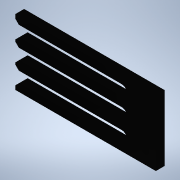
# Autodesk Inventor part: SampleMountFingers
Saved by Autodesk Inventor 2022.2 (Build 262287000, 287)
## iProperties
Created: 2021-09-07
Part Number: SampleMountFingers
Material: Aluminum 6061
Document SubType Name: Modeling
Designer: Timo
Density: 2.7 g/cm^3
Appearance: Anodized - Black
Author: Timo
Autodesk Inventor part; units mm, degrees
ref_plane "YZ Plane" through (0, 0, 0) normal (1, 0, 0) x (0, 1, 0)
ref_plane "XZ Plane" through (0, 0, 0) normal (0, 1, 0) x (-1, 0, 0)
ref_plane "XY Plane" through (0, 0, 0) normal (0, 0, 1) x (1, 0, 0)
sketch "Sketch1" plane through (0, 0, 0) normal (0, 0, 1) x (1, 0, 0)
  line L0 (0, 0) -> (-60, 0) construction
  line L1 (0, 3.1) -> (-60, 3.1)
  line L2 (-60, -3.1) -> (0, -3.1)
  arc A0 (0, -3.1) -> (0, 3.1) centre (0, 0) ccw
  arc A1 (-60, 3.1) -> (-60, -3.1) centre (-60, 0) ccw
  line L3 (0, 11.2) -> (-60, 11.2) construction
  line L4 (0, 14.3) -> (-60, 14.3)
  line L5 (-60, 8.1) -> (0, 8.1)
  arc A2 (0, 8.1) -> (0, 14.3) centre (0, 11.2) ccw
  arc A3 (-60, 14.3) -> (-60, 8.1) centre (-60, 11.2) ccw
  line L6 (0, -11.2) -> (-60, -11.2) construction
  line L7 (0, -8.1) -> (-60, -8.1)
  line L8 (-60, -14.3) -> (0, -14.3)
  arc A4 (0, -14.3) -> (0, -8.1) centre (0, -11.2) ccw
  arc A5 (-60, -8.1) -> (-60, -14.3) centre (-60, -11.2) ccw
  line L9 (7.3, -3.9) -> (-7.3, -3.9) construction
  line L10 (-7.3, -3.9) -> (-7.3, -18.5) construction
  line L11 (-7.3, -18.5) -> (7.3, -18.5) construction
  line L12 (7.3, -18.5) -> (7.3, -3.9) construction
  line L13 (7.3, 3.9) -> (-7.3, 3.9) construction
  line L14 (-7.3, 3.9) -> (-7.3, 18.5) construction
  line L15 (-7.3, 18.5) -> (7.3, 18.5) construction
  line L16 (7.3, 18.5) -> (7.3, 3.9) construction
  line L17 (-7.3, -3.9) -> (7.3, -18.5) construction
  line L18 (7.3, -3.9) -> (-7.3, -18.5) construction
  line L19 (-7.3, 18.5) -> (7.3, 3.9) construction
  line L20 (7.3, 18.5) -> (-7.3, 3.9) construction
  line L21 (0, -25.9) -> (0, 25.9) construction
  line L22 (-60, 18.5) -> (7.3, 18.5)
  line L23 (7.3, 18.5) -> (7.3, -18.5)
  line L24 (7.3, -18.5) -> (-60, -18.5)
  line L25 (-60, -18.5) -> (-60, 18.5)
  line L26 (7.3, 18.5) -> (19.3, 18.5)
  line L27 (19.3, 18.5) -> (19.3, -18.5)
  line L28 (19.3, -18.5) -> (7.3, -18.5)
  line L29 (7.3, -18.5) -> (7.3, 18.5)
  point P0 (-30, 0)
  point P1 (-30, 11.2)
  point P2 (-30, -11.2)
  point P3 (0, -11.2)
  dimension "d0" = 6.2
  dimension "d1" = 14.6
  dimension "d2" = 14.6
  dimension "d5" = 60
  dimension "d11" = 11.2
  dimension "d12" = 5
  dimension "d13" = 5
  dimension "d17" = 37
  dimension "d18" = 12
  constraints: 64 end point, 13 parallel, 12 point on circle, 12 tangent, 6 centre point, 6 midpoint, 5 horizontal, 5 perpendicular, 4 equal length, 3 point on line, 2 equal radius
  measures "d0" diameter of A1
  measures "d1" distance of L11.end L10.end
  measures "d2" distance of L10.end L9.end
  measures "d5" distance of L6.start L6.end
  measures "d11" distance between parallel lines of L0 L3
  measures "d12" distance between parallel lines of L7 L2
  measures "d13" distance between parallel lines of L1 L5
  measures "d17" distance of L15.end L11.end
  measures "d18" distance of L15.end L26.end
extrude "Extrusion1" add sketch "Sketch1" along normal blind 5 contours L1 L25 L5 A2 L4 L22 L23 L24 L8 A4 L7 L2 A0 | L26 L27 L28 L23
chamfer "Chamfer1" distance 2 angle 45 6 edges at (-60, 14.3, 2.5) (-60, 8.1, 2.5) (-60, 3.1, 2.5) (-60, -3.1, 2.5) (-60, -8.1, 2.5) (-60, -14.3, 2.5)
sketch "Sketch3" plane through (0, 0, 0) normal (0, 0, -1) x (-1, 0, 0)
  line L0 (-19.3, 18.5) -> (-7.3, 18.5) construction
  line L1 (-7.3, 18.5) -> (-7.3, -18.5) construction
  line L2 (-7.3, -18.5) -> (-19.3, -18.5) construction
  line L3 (-19.3, -18.5) -> (-19.3, 18.5) construction
  line L4 (60, -18.5) -> (-19.3, -18.5) construction
  line L5 (-19.3, 18.5) -> (60, 18.5) construction
  line L6 (-13.3, 18.5) -> (-13.3, -18.5) construction
  line L7 (60, -18.5) -> (-19.3, -18.5) construction
  line L8 (75.86, 0) -> (-35.16, 0) construction
  point P0 (0, 0)
  point P1 (-13.3, 11.2)
  point P2 (-13.3, -11.2)
  point P3 (-13.3, 0)
  dimension "d19" = 12
  dimension "d20" = 6
  dimension "d21" = 22.4
  dimension "d22" = 37
  constraints: 10 end point, 6 point on line, 2 parallel, 2 perpendicular, 1 horizontal, 1 midpoint, 1 symmetric about line
  measures "d19" distance of L0.start L0.end
  measures "d20" distance between parallel lines of L6 L1
  measures "d21" distance of point (-13.3, 11.2) point (-13.3, -11.2)
  measures "d22" distance of L2.end L0.start
hole "Hole1" at (13.3, 11.2, 0) at (13.3, -11.2, 0) at (13.3, 0, 0) direction (0, 0, 1) diameter 4.2 end through all
equation "\"d2\" = d1"
equation "\"d13\" = d12"
equation "\"d20\" = 0.5 * d19"
body "Solid1"
